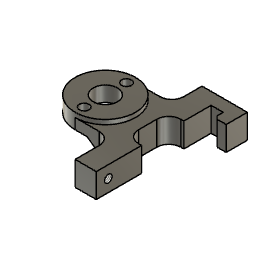
headcamera_arm2 (Autodesk Fusion 360 design; units mm, degrees)
Autodesk Fusion 360 part; units mm, degrees
sketch "スケッチ1" plane through (0, 0, 0) normal (0, 0, 1) x (1, 0, 0)
  circle A0 centre (0, 0) radius 10
  line L0 (0, 10) -> (12, 10)
  line L1 (12, 10) -> (12, 20)
  line L2 (12, 20) -> (27, 20)
  line L3 (27, 20) -> (27, 13)
  line L4 (27, 13) -> (23, 13)
  line L5 (23, 13) -> (23, 16)
  line L6 (23, 16) -> (19, 16)
  line L7 (19, 16) -> (19, -22)
  line L8 (19, -22) -> (12, -22)
  line L9 (12, -22) -> (12, -10)
  line L10 (12, -10) -> (0, -10)
  line L11 (0, -7) -> (0, 7)
  line L12 (19, -7) -> (14, -7)
  line L13 (14, -7) -> (14, 7)
  line L14 (14, 7) -> (19, 7)
  point P0 (14, 0)
  dimension "d1" = 20
  dimension "d2" = 12
  dimension "d4" = 4
  dimension "d5" = 4
  dimension "d6" = 7
  dimension "d8" = 4
  dimension "d9" = 3
  dimension "d19" = 14
  dimension "d29" = 13
  dimension "d30" = 22
  dimension "d31" = 5
  dimension "d32" = 14
  constraint coincident A0.centre origin
  constraint coincident A0 L0.start
  constraint horizontal L0
  constraint perpendicular L0 L1
  constraint perpendicular L1 L2
  constraint perpendicular L2 L3
  constraint perpendicular L1 L4
  constraint perpendicular L4 L5
  constraint perpendicular L1 L6
  constraint perpendicular L6 L7
  constraint perpendicular L7 L8
  constraint perpendicular L8 L9
  constraint coincident A0 L10.end
  constraint perpendicular L7 L10
  constraint tangent A0 L0
  constraint tangent A0 L10
  constraint collinear L1 L9
  constraint midpoint A0.centre L11
  constraint vertical L11
  constraint coincident L7 L12.start
  constraint perpendicular L7 L12
  constraint perpendicular L12 L13
  constraint coincident L7 L14.end
  constraint perpendicular L7 L14
  constraint midpoint L13 P0
  constraint horizontal A0.centre P0
  measures "d1" diameter of A0
  measures "d2" distance of A0.centre L1
  measures "d4" distance of L3.end L4.end
  measures "d5" distance of L5 L7
  measures "d6" distance of L1 L7
  measures "d8" distance of L2 L6
  measures "d9" distance of L4 L6
  measures "d19" distance of L11.start L11.end
  measures "d29" distance of A0.centre L4
  measures "d30" distance of A0.centre L8
  measures "d31" distance of L12.start L12.end
  measures "d32" distance of L12 L14
extrude "押し出し1" add sketch "スケッチ1" along normal blind 8 contours A0 | A0 L0 L1 L2 L3 L4 L5 L6 L7 L8 L9 L10 L12 L13 L14
sketch "スケッチ2" plane through (0, 0, 8) normal (0, 0, 1) x (-1, 0, 0)
  arc A0 (0, -10) -> (0, 10) centre (0, 0) ccw
  line L0 (0, 10) -> (-12, 10)
  line L1 (-12, 10) -> (-12, 22)
  line L2 (-12, 22) -> (-19, 22)
  line L3 (-19, -7) -> (-19, -16)
  line L4 (-19, -16) -> (-23, -16)
  line L5 (-23, -16) -> (-23, -13)
  line L6 (-23, -13) -> (-27, -13)
  line L7 (-27, -13) -> (-27, -20)
  line L8 (-27, -20) -> (-12, -20)
  line L9 (-12, -20) -> (-12, -10)
  line L10 (-12, -10) -> (0, -10)
  circle A1 centre (0, 0) radius 10
  line L11 (-19, 7) -> (-14, 7)
  line L12 (-14, 7) -> (-14, -7)
  line L13 (-14, -7) -> (-19, -7)
  line L14 (-19, 22) -> (-19, 7)
  constraint concentric A0 A1
extrude "押し出し2" add sketch "スケッチ2" along normal blind 1.5 contours A0 A1
hole "穴1" at (0, 7, 0) at (0, -7, 0) direction (0, 0, 1) diameter 3.2 end through all
hole "穴3" at (0, 0, 0) direction (0, 0, 1) diameter 8 end through all
sketch "スケッチ3" plane through (0, -10, 0) normal (0, -1, 0) x (1, 0, 0)
  line L0 (0, 0) -> (12, 0)
  line L1 (12, 0) -> (12, 8)
  line L2 (12, 8) -> (0, 8)
  line L3 (0, 8) -> (0, 0)
  line L4 (10, 0) -> (4, 4.5)
  line L5 (4, 4.5) -> (-15, 4.5)
  line L6 (-15, 4.5) -> (-15, 0)
  line L7 (-15, 0) -> (10, 0)
  dimension "d20" = 10
  dimension "d21" = 15
  dimension "d22" = 6
  dimension "d23" = 4.5
  constraint coincident L0 L4.start
  constraint parallel L0 L5
  constraint perpendicular L5 L6
  constraint perpendicular L6 L7
  measures "d20" distance of L0.start L4.start
  measures "d21" distance of L0.start L6
  measures "d22" horizontal distance of L4.start L4.end
  measures "d23" vertical distance of L4.start L4.end
extrude "押し出し3" cut sketch "スケッチ3" against normal through all contours L0 L3 L4 L5 L7 | L3 L5 L6 L7
sketch "スケッチ4" plane through (19, 0, 0) normal (1, 0, 0) x (0, 1, 0)
  line L0 (-22, 0) -> (-7, 0)
  line L1 (16, 0) -> (16, 8)
  line L2 (-7, 8) -> (-22, 8)
  line L3 (-22, 8) -> (-22, 0)
  line L4 (-22, 4) -> (-18, 4)
  line L5 (-7, 0) -> (-7, 8)
  line L6 (7, 0) -> (16, 0)
  line L7 (16, 8) -> (7, 8)
  line L8 (7, 8) -> (7, 0)
  dimension "d25" = 4
  constraint perpendicular L3 L4
  constraint midpoint L3 L4.start
  measures "d25" distance of L4.start L4.end
hole "穴2" at (19, -18, 4) direction (-1, 0, 0) diameter 3 depth 11 tip angle 118
thread "ねじ1" "ISO Metric profile 3.0 M3x0.5 6H" major diameter 3.086 minor diameter 2.529 pitch 0.5 angle 60 resizes the face on face at (16.6667, -17.8506, 5.4925)
chamfer "面取り1" distance 1 angle 45 1 edges at (23, 13, 4)
fillet "フィレット1" radius 4 4 edges at (12, 10, 4) (12, -10, 4) (14, -7, 4) (14, 7, 4)
